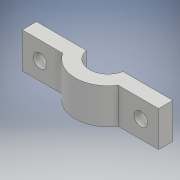
# Autodesk Inventor part: twoscrewclamp
Saved by Autodesk Inventor 2018 (Build 220112000, 112)
## iProperties
Created: 2018-11-04
Part Number: twoscrewclamp
Material: Generic
Document SubType Name: Modeling
Designer: Prakash
Density: 1 g/cm^3
Appearance: Default
Author: Prakash
Autodesk Inventor part; units mm, degrees
ref_plane "YZ Plane" through (0, 0, 0) normal (1, 0, 0) x (0, 1, 0)
ref_plane "XZ Plane" through (0, 0, 0) normal (0, 1, 0) x (-1, 0, 0)
ref_plane "XY Plane" through (0, 0, 0) normal (0, 0, 1) x (1, 0, 0)
sketch "Sketch1" plane through (0, 0, 0) normal (0, 0, 1) x (1, 0, 0)
  line L0 (0, 0) -> (14, 0)
  arc A0 (14, 0) -> (24.3078, 0) centre (19.1539, 1) ccw
  line L1 (24.3078, 0) -> (38.3078, 0)
  line L2 (19.1539, 0) -> (19.1539, 1) construction
  line L3 (14, 0) -> (19.1539, 0) construction
  line L4 (24.3078, 0) -> (19.1539, 0) construction
  line L5 (0, 0) -> (0, -4)
  arc A1 (11.3717, -4) -> (26.9361, -4) centre (19.1539, 1) ccw
  line L6 (0, -4) -> (11.3717, -4)
  line L7 (38.3078, 0) -> (38.3078, -4)
  line L8 (38.3078, -4) -> (26.9361, -4)
  dimension "d0" = 14
  dimension "d2" = 10.5
  dimension "d3" = 14
  dimension "d4" = 1
  dimension "d6" = 4
  dimension "d7" = 18.5
  dimension "d8" = 4
  constraints: 18 end point, 4 horizontal, 4 point on circle, 3 collinear, 3 vertical, 2 centre point, 1 coincident
  measures "d0" distance of L0.start L0.end
  measures "d2" diameter of A0
  measures "d3" distance of L1.start L1.end
  measures "d4" distance of L2.start L2.end
  measures "d6" distance of L0.start L5.end
  measures "d7" diameter of A1
  measures "d8" distance of L1.end L7.end
extrude "Extrusion1" add sketch "Sketch1" along normal blind 10
sketch "Sketch9" plane through (0, 0, 10) normal (0, 1, 0) x (1, 0, 0)
  line L0 (14, 0) -> (0, 0) projected
  line L1 (0, 10) -> (10, 10)
  line L2 (10, 10) -> (10, 0)
  line L3 (10, 0) -> (0, 0)
  line L4 (0, 0) -> (0, 10)
  line L5 (24.3078, 10) -> (38.3078, 10) projected
  line L6 (38.3078, 0) -> (24.3078, 0) projected
  line L7 (38.3287, 10) -> (28.3287, 10)
  line L8 (28.3287, 10) -> (28.3287, 0)
  line L9 (28.3287, 0) -> (38.3287, 0)
  line L10 (38.3287, 0) -> (38.3287, 10)
  line L11 (0, 0) -> (10, 10) construction
  line L12 (0, 10) -> (0, 0) projected
  line L13 (0, 10) -> (10, 0) construction
  line L14 (28.3287, 0) -> (38.3287, 10) construction
  line L15 (38.3287, 0) -> (28.3287, 10) construction
  line L16 (48.3078, 0) -> (38.3287, 0)
  line L17 (38.3287, 0) -> (38.3287, 10)
  line L18 (38.3287, 10) -> (48.3078, 10)
  line L19 (48.3078, 10) -> (48.3078, 0)
  line L20 (48.3078, 10) -> (48.3078, 0) projected
  line L21 (48.3078, 10) -> (38.3287, 0) construction
  line L22 (48.3078, 0) -> (38.3287, 10) construction
  point P0 (28.3497, 10)
  point P1 (5, 5)
  point P2 (33.3287, 5)
  point P3 (43.3182, 5)
  dimension "d38" = 10
  dimension "d39" = 10
  constraints: 36 end point, 6 parallel, 5 perpendicular, 5 point on line, 3 horizontal, 3 midpoint
  measures "d38" distance of L2.end L3.end
  measures "d39" distance of L9.end L8.end
hole "Hole1" at (5, 0, 5) at (33.3287, 0, 5) at (43.3182, 0, 5) direction (0, -1, 0) diameter 3.797 end through all clearance for "Flat Head Machine Screw (82)" size "#6" standard "Ansi Unified Screw Threads"
body "Solid1"
